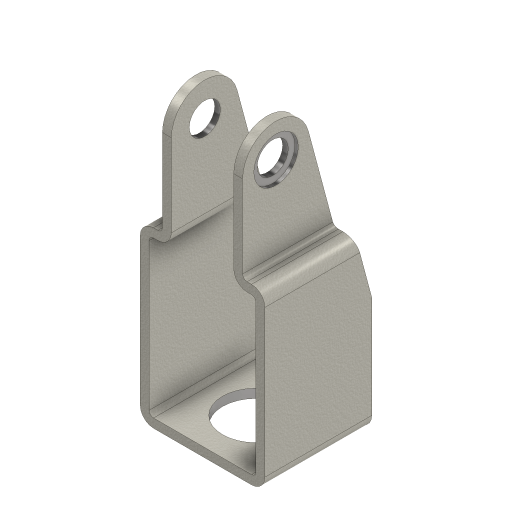
# Autodesk Inventor part: Part021. High fork
Saved by Autodesk Inventor 2023.2 (Build 272271030, 271C)
## iProperties
Created: 2023-09-20
Part Number: Part021. High fork
Material: Steel, Carbon
Document SubType Name: Modeling
Designer: User
Density: 7.85 g/cm^3
Appearance: Steel - Cast
Author: User
Autodesk Inventor part; units mm, degrees
ref_plane "YZ Plane" through (0, 0, 0) normal (1, 0, 0) x (0, 1, 0)
ref_plane "XZ Plane" through (0, 0, 0) normal (0, 1, 0) x (-1, 0, 0)
ref_plane "XY Plane" through (0, 0, 0) normal (0, 0, 1) x (1, 0, 0)
sketch "Sketch1" plane through (0, 0, 0) normal (0, 0, 1) x (1, 0, 0)
  line L0 (-18, 132) -> (-18, 80)
  line L1 (-20, 78) -> (-22, 78)
  line L2 (-28, 72) -> (-28, 6)
  line L3 (-22, 0) -> (22, 0)
  line L4 (28, 6) -> (28, 72)
  line L5 (22, 78) -> (20, 78)
  line L6 (18, 80) -> (18, 132)
  arc A0 (-28, 6) -> (-22, 0) centre (-22, 6) ccw
  arc A1 (-22, 78) -> (-28, 72) centre (-22, 72) ccw
  arc A2 (28, 72) -> (22, 78) centre (22, 72) ccw
  arc A3 (22, 0) -> (28, 6) centre (22, 6) ccw
  arc A4 (-20, 78) -> (-18, 80) centre (-20, 80) ccw
  arc A5 (18, 80) -> (20, 78) centre (20, 80) ccw
  line L7 (-14, 132) -> (-14, 80)
  arc A6 (-20, 74) -> (-14, 80) centre (-20, 80) ccw
  line L8 (-20, 74) -> (-22, 74)
  arc A7 (-22, 74) -> (-24, 72) centre (-22, 72) ccw
  line L9 (-24, 72) -> (-24, 6)
  arc A8 (-24, 6) -> (-22, 4) centre (-22, 6) ccw
  line L10 (-22, 4) -> (22, 4)
  arc A9 (22, 4) -> (24, 6) centre (22, 6) ccw
  line L11 (24, 6) -> (24, 72)
  arc A10 (24, 72) -> (22, 74) centre (22, 72) ccw
  line L12 (22, 74) -> (20, 74)
  arc A11 (14, 80) -> (20, 74) centre (20, 80) ccw
  line L13 (14, 80) -> (14, 132)
  line L14 (14, 132) -> (18, 132)
  line L15 (-14, 132) -> (-18, 132)
  point P0 (0, 0)
  point P1 (0, 0)
  dimension "d0" = 132
  dimension "d1" = 6
  dimension "d2" = 2
  dimension "d3" = 56
  dimension "d4" = 36
  dimension "d5" = 4
  dimension "d6" = 78
  constraints: 32 end point, 24 point on circle, 12 centre point, 12 perpendicular, 12 tangent, 4 equal radius, 3 equal length, 1 coincident, 1 collinear, 1 horizontal, 1 midpoint, 1 vertical, 12 other
  measures "d0" distance from line of L3 L0.start
  measures "d1" radius of A0
  measures "d2" radius of A4
  measures "d3" distance between parallel lines of L4 L2
  measures "d4" distance between parallel lines of L6 L0
  measures "d5" distance between parallel lines of L0 L7
  measures "d6" distance between parallel lines of L3 L1
extrude "Extrusion1" add sketch "Sketch1" along normal blind 15 and the other way blind 33
fillet "Fillet1" radius 15 2 edges at (-16, 132, 15) (16, 132, 15)
sketch "Sketch3" plane through (0, 0, 0) normal (1, 0, 0) x (0, 1, 0)
  arc A0 (132, 0) -> (117, 15) centre (117, 0) ccw projected
  line L0 (72, -33) -> (6, -33) projected
  arc A1 (120.8823, -14.4889) -> (132, 0) centre (117, 0) ccw
  line L1 (120.8823, -14.4889) -> (51.7979, -33)
  line L2 (6, 15) -> (72, 15) projected
  line L3 (51.7979, -33) -> (132, -33)
  line L4 (132, -33) -> (132, 0) projected
  point P0 (0, 0)
  dimension "d12" = 15
  constraints: 4 end point, 3 point on circle, 1 centre point, 1 coincident, 1 horizontal, 1 point on line, 1 tangent
  measures "d12" angle of L1 L2
extrude "Extrusion2" cut sketch "Sketch3" along normal through all both and the other way through all
sketch "Sketch4" plane through (18, 80, 15) normal (1, 0, 0) x (0, 0, -1)
  arc A0 (29.4889, 40.8823) -> (0, 37) centre (15, 37) ccw projected
  point P0 (15, -80)
  constraints: 1 coincident
hole "Hole1" at (18, 117, 0) direction (-1, 0, 0) diameter 14 depth 4 counterbore diameter 20 counterbore depth 1.5
mirror "Mirror1" about plane through (0, 0, 0) normal (1, 0, 0) of "Hole1"
sketch "Sketch5" plane through (-22, 4, 15) normal (0, 1, 0) x (1, 0, 0)
  line L0 (44, 48) -> (0, 0)
  point P0 (22, 15)
  point P1 (22, 24)
  constraints: 2 end point, 1 midpoint
hole "Hole2" at (0, 4, -9) direction (0, -1, 0) diameter 30 end through all
body "Solid1"
